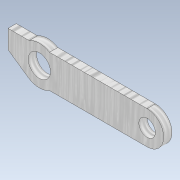
# Autodesk Inventor part: アーム揺動節test
Saved by Autodesk Inventor 2020.3 (Build 243373000, 373)
## iProperties
Created: 2020-02-28
Part Number: アーム揺動節test
Material: アルミニウム 7075
Document SubType Name: Modeling
Designer: aoyam
Density: 2.81 g/cm^3
Appearance: サテン - ブラシ仕上げ 重厚
Mass: 4.89311 g
Surface Area: 18.0863 cm^2
Volume: 1.74132 cm^3
Author: aoyam
Autodesk Inventor part; units mm, degrees
ref_plane "YZ Plane" through (0, 0, 0) normal (1, 0, 0) x (0, 1, 0)
ref_plane "XZ Plane" through (0, 0, 0) normal (0, 1, 0) x (-1, 0, 0)
ref_plane "XY Plane" through (0, 0, 0) normal (0, 0, 1) x (1, 0, 0)
sketch "スケッチ1" plane through (0, 0, 0) normal (0, 0, 1) x (1, 0, 0)
  line L0 (0, 0) -> (-39, 0)
  circle A0 centre (-39, 0) radius 4.025
  circle A1 centre (0, 0) radius 2.99
  circle A2 centre (-39, 0) radius 7.025
  circle A3 centre (0, 0) radius 5.99
  line L1 (-46.025, 5.99) -> (5.99, 5.99)
  line L2 (5.99, 5.99) -> (5.99, -5.99)
  line L3 (5.99, -5.99) -> (-46.025, -5.99)
  line L4 (-46.025, -5.99) -> (-46.025, 5.99)
  line L5 (-46.025, 5.99) -> (-60, 5.99)
  line L6 (-60, 5.99) -> (-42.9977, -5.7766)
  line L7 (-50.3367, 5.99) -> (-50.3367, -0.6976)
  point P0 (-35.3298, -5.99)
  point P1 (-35.3298, 5.99)
  point P2 (0, 5.99)
  point P3 (0, -5.99)
  point P4 (-29.6595, 5.99)
  point P5 (-42.6702, 5.99)
  point P6 (-40.3405, 5.99)
  point P7 (-40.3405, -5.99)
  point P8 (-42.6702, -5.99)
  point P9 (-29.6595, -5.99)
  point P10 (-46.025, 0)
  point P11 (5.99, 0)
  point P12 (-46.025, -3.6815)
  dimension "d0" = 39
  dimension "d1" = 8.05
  dimension "d2" = 5.98
  dimension "d3" = 3
  dimension "d4" = 3
  constraints: 16 end point, 3 centre point, 3 horizontal, 3 tangent, 2 coincident, 2 parallel, 2 point on line, 2 vertical, 1 perpendicular, 4 other
  measures "d0" distance of L0.start L0.end
  measures "d1" diameter of A0
  measures "d2" diameter of A1
  measures "d4" radial gap between concentric circles of A1 A3
extrude "押し出し1" add sketch "スケッチ1" along normal blind 3 contours A2 L1 A3 L0 | A2 L3 L1 | L0 A3 L3 A2 | A3 | L1 A2 | A2 L3 | A2 L4 L1 | A2 L6 L4 | L4 L6 L7 L5
sketch "スケッチ2" plane through (0, 0, 0) normal (0, 0, -1) x (-1, 0, 0)
  arc A0 (35.3298, -5.99) -> (42.9977, -5.7766) centre (39, 0) ccw projected
  line L0 (50.3367, -0.6976) -> (42.9977, -5.7766) projected
  line L1 (50.3367, 5.99) -> (50.3367, -0.6976) projected
  line L2 (42.6702, 5.99) -> (50.3367, 5.99) projected
  arc A1 (42.6702, 5.99) -> (35.3298, 5.99) centre (39, 0) ccw projected
  line L3 (0, 5.99) -> (35.3298, 5.99) projected
  arc A2 (0, 5.99) -> (0, -5.99) centre (0, 0) ccw projected
  line L4 (35.3298, -5.99) -> (0, -5.99) projected
  circle A3 centre (39, 0) radius 4.025 projected
  circle A4 centre (0, 0) radius 2.99 projected
  line L5 (47.026, -2.9887) -> (48.56, -0.3319) construction
  line L6 (47.9354, -3.5137) -> (49.4693, -0.8569)
  line L7 (47.6506, 0.1931) -> (46.1167, -2.4637)
  arc A5 (46.1167, -2.4637) -> (47.9354, -3.5137) centre (47.026, -2.9887) ccw
  arc A6 (49.4693, -0.8569) -> (47.6506, 0.1931) centre (48.56, -0.3319) ccw
  point P0 (47.793, -1.6603)
  point P1 (46.1626, -3.5863)
  point P2 (49.0453, -1.5913)
  dimension "d11" = 2.1
  dimension "d12" = 30
  constraints: 8 end point, 4 point on circle, 4 tangent, 2 centre point, 1 midpoint, 1 parallel, 1 point on line, 1 other
  measures "d11" diameter of A6
  measures "d12" angle of L5 L1
